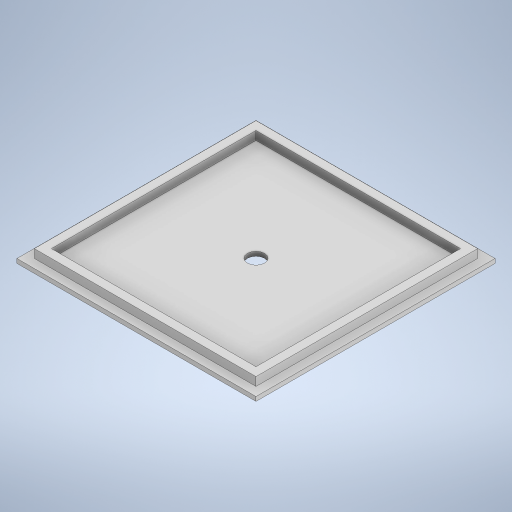
# Autodesk Inventor part: base-lid
Saved by Autodesk Inventor 2024 (Build 280153000, 153)
## iProperties
Created: 2024-01-23
Part Number: base-lid
Material: Generic
Document SubType Name: Modeling
Designer: emosh
Density: 1 g/cm^3
Appearance: Default
Author: emosh
## iProperties of the stored document base-lid_3DPrint.ipt
Created: 2024-01-24
Part Number: base-lid_3DPrint
Material: Generic
Document SubType Name: Modeling
Designer: emosh
Density: 1 g/cm^3
Appearance: Default
Author: emosh
Autodesk Inventor part; units mm, degrees
ref_plane "YZ Plane" through (0, 0, 0) normal (1, 0, 0) x (0, 1, 0)
ref_plane "XZ Plane" through (0, 0, 0) normal (0, 1, 0) x (-1, 0, 0)
ref_plane "XY Plane" through (0, 0, 0) normal (0, 0, 1) x (1, 0, 0)
sketch "Sketch7" plane through (0, 0, 0) normal (0, 1, 0) x (-1, 0, 0)
  line L0 (0, 0) -> (177.8, 0)
  line L1 (177.8, 0) -> (177.8, -177.8)
  line L2 (177.8, -177.8) -> (0, -177.8)
  line L3 (0, -177.8) -> (0, 0)
  dimension "d29" = 177.8
  dimension "d30" = 177.8
  constraints: 8 end point, 2 parallel, 1 horizontal, 1 perpendicular
  measures "d29" distance of L1.end L2.end
  measures "d30" distance of L0.end L1.end
extrude "Extrusion6" add sketch "Sketch7" along normal blind 3.175
sketch "Sketch8" plane through (0, 3.175, 0) normal (0, 1, 0) x (1, 0, 0)
  line L0 (-177.8, 0) -> (0, 0) projected
  line L1 (-177.8, 0) -> (-171.323, 0)
  line L2 (-171.323, 0) -> (-171.323, 6.477)
  line L3 (-171.323, 6.477) -> (-177.8, 6.477)
  line L4 (-177.8, 6.477) -> (-177.8, 0)
  line L5 (0, 177.8) -> (-177.8, 177.8) projected
  line L6 (0, 177.8) -> (-6.477, 177.8)
  line L7 (-6.477, 177.8) -> (-6.477, 171.323)
  line L8 (-6.477, 171.323) -> (0, 171.323)
  line L9 (0, 171.323) -> (0, 177.8)
  line L10 (-6.477, 171.323) -> (-171.323, 171.323)
  line L11 (-171.323, 171.323) -> (-171.323, 6.477)
  line L12 (-171.323, 6.477) -> (-6.477, 6.477)
  line L13 (-6.477, 6.477) -> (-6.477, 171.323)
  line L14 (-171.323, 6.477) -> (-164.973, 6.477)
  line L15 (-164.973, 6.477) -> (-164.973, 12.827)
  line L16 (-164.973, 12.827) -> (-171.323, 12.827)
  line L17 (-171.323, 12.827) -> (-171.323, 6.477)
  line L18 (-6.477, 171.323) -> (-12.827, 171.323)
  line L19 (-12.827, 171.323) -> (-12.827, 164.973)
  line L20 (-12.827, 164.973) -> (-6.477, 164.973)
  line L21 (-6.477, 164.973) -> (-6.477, 171.323)
  line L22 (-12.827, 164.973) -> (-164.973, 164.973)
  line L23 (-164.973, 164.973) -> (-164.973, 12.827)
  line L24 (-164.973, 12.827) -> (-12.827, 12.827)
  line L25 (-12.827, 12.827) -> (-12.827, 164.973)
  dimension "d33" = 6.477
  dimension "d34" = 6.477
  dimension "d35" = 6.477
  dimension "d36" = 6.477
  dimension "d37" = 6.35
  dimension "d38" = 6.35
  dimension "d39" = 6.35
  dimension "d40" = 6.35
  constraints: 48 end point, 12 parallel, 6 horizontal, 6 perpendicular
  measures "d33" distance of L3.end L2.end
  measures "d34" distance of L2.end L1.end
  measures "d35" distance of L8.end L7.end
  measures "d36" distance of L7.end L6.end
  measures "d37" distance of L16.end L15.end
  measures "d38" distance of L15.end L14.end
  measures "d39" distance of L20.end L19.end
  measures "d40" distance of L19.end L18.end
extrude "Extrusion7" add sketch "Sketch8" along normal blind 6.35 contours L11 L16 L15 L12 | L11 L10 L19 L22 L23 L16 | L15 L24 L25 L20 L13 L12 | L10 L13 L20 L19
sketch "Sketch9" plane through (0, 3.175, 0) normal (0, 1, 0) x (1, 0, 0)
  line L0 (-164.973, 12.827) -> (-12.827, 12.827) projected
  line L1 (-12.827, 12.827) -> (-89.027, 12.827)
  line L2 (-89.027, 12.827) -> (-89.027, 89.027)
  line L3 (-89.027, 89.027) -> (-12.827, 89.027)
  line L4 (-12.827, 89.027) -> (-12.827, 12.827)
  circle A0 centre (-89.027, 89.027) radius 6.35
  point P0 (0, 0)
  dimension "d43" = 76.2
  dimension "d44" = 76.2
  dimension "d45" = 12.7
  constraints: 8 end point, 2 parallel, 1 centre point, 1 coincident, 1 horizontal, 1 perpendicular
  measures "d43" distance of L2.end L3.end
  measures "d44" distance of L1.end L2.end
  measures "d45" diameter of A0
extrude "Extrusion8" cut sketch "Sketch9" against normal blind 6.35 contours A0 L3 L2 | L2 L3 A0
body "Solid2"
